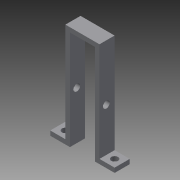
# Autodesk Inventor part: BarClip
Saved by Autodesk Inventor 2014 SP1 (Build 180222100, 222)
## iProperties
Created: 2014-06-21
Part Number: BarClip
Material: Generic
Document SubType Name: Modeling
Designer: Erin
Density: 1 g/cm^3
Appearance: Default
Author: Erin
Autodesk Inventor part; units mm, degrees
ref_plane "YZ Plane" through (0, 0, 0) normal (1, 0, 0) x (0, 1, 0)
ref_plane "XZ Plane" through (0, 0, 0) normal (0, 1, 0) x (-1, 0, 0)
ref_plane "XY Plane" through (0, 0, 0) normal (0, 0, 1) x (1, 0, 0)
sketch "Sketch1" plane through (0, 0, 0) normal (0, 1, 0) x (-1, 0, 0)
  line L0 (-14.3889, -14.2778) -> (-11.3889, -14.2778)
  line L1 (-11.3889, -14.2778) -> (-11.3889, 54.2222)
  line L2 (-11.3889, 54.2222) -> (-14.3889, 54.2222)
  line L3 (-14.3889, 54.2222) -> (-14.3889, -14.2778)
  line L4 (-11.3889, 54.2222) -> (5.1111, 54.2222)
  line L5 (5.1111, 54.2222) -> (5.1111, 51.2222)
  line L6 (5.1111, 51.2222) -> (-11.3889, 51.2222)
  line L7 (-11.3889, 51.2222) -> (-11.3889, 54.2222)
  line L8 (5.1111, 54.2222) -> (8.1111, 54.2222)
  line L9 (8.1111, 54.2222) -> (8.1111, -14.2778)
  line L10 (8.1111, -14.2778) -> (5.1111, -14.2778)
  line L11 (5.1111, -14.2778) -> (5.1111, 54.2222)
  line L12 (8.1111, -14.2778) -> (18.1111, -14.2778)
  line L13 (18.1111, -14.2778) -> (18.1111, -11.2778)
  line L14 (18.1111, -11.2778) -> (8.1111, -11.2778)
  line L15 (8.1111, -11.2778) -> (8.1111, -14.2778)
  line L16 (-14.3889, -14.2778) -> (-24.3889, -14.2778)
  line L17 (-24.3889, -14.2778) -> (-24.3889, -11.2778)
  line L18 (-24.3889, -11.2778) -> (-14.3889, -11.2778)
  line L19 (-14.3889, -11.2778) -> (-14.3889, -14.2778)
  point P0 (0, 0)
  dimension "d0" = 10
  dimension "d1" = 10
  dimension "d2" = 3
  dimension "d3" = 3
  dimension "d4" = 3
  dimension "d5" = 3
  dimension "d6" = 3
  dimension "d7" = 68.5
  dimension "d8" = 16.5
  constraints: 40 end point, 10 parallel, 5 horizontal, 5 perpendicular, 1 collinear
  measures "d0" distance of L0.start L16.end
  measures "d1" distance of L9.end L12.end
  measures "d2" distance of L12.end L13.end
  measures "d3" distance of L16.end L17.end
  measures "d4" distance of L0.start L0.end
  measures "d5" distance of L9.end L10.end
  measures "d6" distance between parallel lines of L6 L4
  measures "d7" distance of L2.end L0.start
  measures "d8" distance between parallel lines of L11 L1
extrude "Extrusion1" add sketch "Sketch1" along normal blind 10
sketch "Sketch2" plane through (14.3889, 0, 54.2222) normal (1, 0, 0) x (0, 0, -1)
  line L0 (0, 10) -> (65.5, 10) projected
  line L1 (0, 0) -> (65.5, 0) projected
  line L2 (31.75, 14.4261) -> (31.75, -5.3494)
  line L3 (68.5, 0) -> (68.5, 10) projected
  circle A0 centre (36.75, 4.5383) radius 2.25
  line L4 (31.75, 4.5383) -> (48.4854, 4.5383)
  point P0 (54.2222, 0)
  dimension "d11" = 36.75
  dimension "d12" = 4.5
  dimension "d13" = 5
  constraints: 4 end point, 1 centre point, 1 midpoint, 1 parallel, 1 perpendicular, 1 point on line
  measures "d11" distance between parallel lines of L2 L3
  measures "d12" diameter of A0
  measures "d13" distance from line of A0.centre L2
extrude "Extrusion2" cut sketch "Sketch2" against normal blind 40
sketch "Sketch3" plane through (14.3889, 0, -11.2778) normal (0, 0, 1) x (1, 0, 0)
  circle A0 centre (5, 5) radius 2.25
  point P0 (-14.3889, 0)
  dimension "d16" = 4.5
  constraints: 1 centre point
  measures "d16" diameter of A0
extrude "Extrusion3" cut sketch "Sketch3" against normal blind 3
sketch "Sketch4" plane through (-18.1111, 0, -11.2778) normal (0, 0, 1) x (1, 0, 0)
  circle A0 centre (5, 5) radius 2.25
  point P0 (18.1111, 0)
  dimension "d19" = 4.5
  constraints: 1 centre point
  measures "d19" diameter of A0
extrude "Extrusion4" cut sketch "Sketch4" against normal blind 3
body "Solid1"
